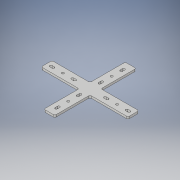
# Autodesk Inventor part: 2
Saved by Autodesk Inventor 2019 (Build 230136000, 136)
## iProperties
Created: 2021-01-29
Part Number: 2
Material: 一般
Document SubType Name: Modeling
Designer: X1 Carbon
Density: 1 g/cm^3
Appearance: 既定
Author: X1 Carbon
Autodesk Inventor part; units mm, degrees
ref_plane "YZ Plane" through (0, 0, 0) normal (1, 0, 0) x (0, 1, 0)
ref_plane "XZ Plane" through (0, 0, 0) normal (0, 1, 0) x (-1, 0, 0)
ref_plane "XY Plane" through (0, 0, 0) normal (0, 0, 1) x (1, 0, 0)
sketch "スケッチ1" plane through (0, 0, 0) normal (0, 1, 0) x (-1, 0, 0)
  circle A0 centre (0, -15) radius 1.65
  circle A1 centre (0, -13.35) radius 1.65
  circle A2 centre (0, -16.65) radius 1.65
  line L0 (1.65, -13.35) -> (1.65, -16.65)
  line L1 (-1.65, -13.35) -> (-1.65, -16.65)
  circle A3 centre (0, -30) radius 1.65
  circle A4 centre (0, -45) radius 1.65
  circle A5 centre (0, -46.65) radius 1.65
  circle A6 centre (0, -43.35) radius 1.65
  line L2 (-1.65, -46.65) -> (-1.65, -43.35)
  line L3 (1.65, -46.65) -> (1.65, -43.35)
  circle A7 centre (-22.5, 0) radius 1.65
  circle A8 centre (-20.85, 0) radius 1.65
  circle A9 centre (-24.15, 0) radius 1.65
  line L4 (-20.85, -1.65) -> (-24.15, -1.65)
  line L5 (-24.15, 1.65) -> (-20.85, 1.65)
  circle A10 centre (-37.5, 0) radius 1.65
  circle A11 centre (-52.5, 0) radius 1.65
  circle A12 centre (-54.15, 0) radius 1.65
  circle A13 centre (-50.85, 0) radius 1.65
  line L6 (-50.85, -1.65) -> (-54.15, -1.65)
  line L7 (-50.85, 1.65) -> (-54.15, 1.65)
  circle A14 centre (0, 30) radius 1.65
  circle A15 centre (37.5, 0) radius 1.65
  circle A16 centre (22.5, 0) radius 1.65
  circle A17 centre (24.15, 0) radius 1.65
  circle A18 centre (20.85, 0) radius 1.65
  line L8 (24.15, -1.65) -> (20.85, -1.65)
  line L9 (20.85, 1.65) -> (24.15, 1.65)
  circle A19 centre (52.5, 0) radius 1.65
  circle A20 centre (54.15, 0) radius 1.65
  circle A21 centre (50.85, 0) radius 1.65
  line L10 (54.15, -1.65) -> (50.85, -1.65)
  line L11 (54.15, 1.65) -> (50.85, 1.65)
  circle A22 centre (0, 15) radius 1.65
  circle A23 centre (0, 13.35) radius 1.65
  circle A24 centre (0, 16.65) radius 1.65
  circle A25 centre (0, 45) radius 1.65
  circle A26 centre (0, 43.35) radius 1.65
  circle A27 centre (0, 46.65) radius 1.65
  line L12 (1.65, 43.35) -> (1.65, 46.65)
  line L13 (-1.65, 43.35) -> (-1.65, 46.65)
  line L14 (-60, -7.5) -> (60, -7.5)
  line L15 (60, -7.5) -> (60, 7.5)
  line L16 (60, 7.5) -> (-60, 7.5)
  line L17 (-60, 7.5) -> (-60, -7.5)
  line L18 (-60, -7.5) -> (60, 7.5) construction
  line L19 (60, -7.5) -> (-60, 7.5) construction
  line L20 (7.5, -56.25) -> (7.5, 56.25)
  line L21 (7.5, 56.25) -> (-7.5, 56.25)
  line L22 (-7.5, 56.25) -> (-7.5, -56.25)
  line L23 (-7.5, -56.25) -> (7.5, -56.25)
  line L24 (7.5, -56.25) -> (-7.5, 56.25) construction
  line L25 (7.5, 56.25) -> (-7.5, -56.25) construction
  line L26 (-1.65, 13.354) -> (-1.65, 16.65)
  line L27 (1.65, 16.65) -> (1.65, 13.35)
  point P0 (0, 0)
  point P1 (0, 0)
  dimension "d0" = 3.3
  dimension "d1" = 3.3
  dimension "d2" = 3.3
  dimension "d3" = 3.3
  dimension "d4" = 3.3
  dimension "d5" = 3.3
  dimension "d6" = 3.3
  dimension "d7" = 3.3
  dimension "d8" = 3.3
  dimension "d9" = 3.3
  dimension "d10" = 3.3
  dimension "d11" = 3.3
  dimension "d12" = 3.3
  dimension "d17" = 120
  dimension "d18" = 15
  dimension "d19" = 112.5
  dimension "d20" = 15
  constraints: 62 point on circle, 56 end point, 28 centre point, 17 tangent, 12 coincident, 9 parallel, 4 midpoint, 3 horizontal, 3 vertical, 2 perpendicular
  measures "d0" diameter of A0
  measures "d1" diameter of A3
  measures "d2" diameter of A4
  measures "d3" diameter of A7
  measures "d4" diameter of A10
  measures "d5" diameter of A11
  measures "d6" diameter of A14
  measures "d7" diameter of A15
  measures "d8" diameter of A16
  measures "d9" diameter of A17
  measures "d10" diameter of A19
  measures "d11" diameter of A22
  measures "d12" diameter of A25
  measures "d17" distance of L14.start L14.end
  measures "d18" distance of L15.end L14.end
  measures "d19" distance of L20.start L20.end
  measures "d20" distance of L21.end L20.end
extrude "押し出し2" add sketch "スケッチ1" along normal blind 3
fillet "フィレット2" radius 2 12 edges at (60, 1.5, -7.5) (60, 1.5, 7.5) (7.5, 1.5, 56.25) (-7.5, 1.5, 56.25) (-60, 1.5, 7.5) (-60, 1.5, -7.5) (-7.5, 1.5, -56.25) (7.5, 1.5, -56.25) (-7.5, 1.5, 7.5) (-7.5, 1.5, -7.5) (7.5, 1.5, 7.5) (7.5, 1.5, -7.5)
